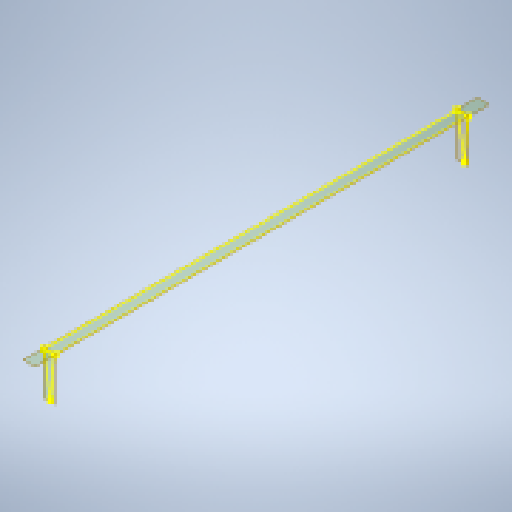
# Autodesk Inventor part: Aleiron
Saved by Autodesk Inventor 2026 (Build 300175050, 175E)
## iProperties
Created: 2025-07-28
Part Number: Aleiron
Material: Generic
Document SubType Name: Modeling
Designer: Cupri
Density: 1 g/cm^3
Appearance: Default
Author: Cupri
Autodesk Inventor part; units mm, degrees
ref_plane "YZ Plane" through (0, 0, 0) normal (1, 0, 0) x (0, 1, 0)
ref_plane "XZ Plane" through (0, 0, 0) normal (0, 1, 0) x (-1, 0, 0)
ref_plane "Work Plane1" through (0, 0, 0) normal (0, 0, 1) x (1, 0, 0)
sketch "Sketch1" plane through (0, 0, 0) normal (0, 0, 1) x (1, 0, 0)
  spline S0 degree 3 poles (-0.3432, 0) (-0.5476, 0.9305) (-1.8109, 6.8833) (-4.6379, 21.5083) (-5.8348, 28.0065) (-7.2785, 36.223) (-7.5554, 37.8163) (-8.144, 41.2441) (-8.4751, 43.1968) (-9.6001, 49.9214) (-10.403, 54.896) (-11.194, 60) knots -7.723672 -7.723672 -7.723672 -7.723672 -4.852573 -4.852573 -2.692004 -2.692004 -2.185384 -2.185384 -1.605169 -1.605169 -0.053083 -0.053083 -0.053083 -0.053083 projected
  spline S1 degree 3 poles (-0.3324, -0.0487) (-0.3358, -0.0335) (-0.3394, -0.0172) (-0.3432, 0) knots -0.056243 -0.056243 -0.056243 -0.056243 -0.050014 -0.050014 -0.050014 -0.050014 projected
  spline S2 degree 3 poles (0.4003, 0) (0.3914, -0.0334) (0.3779, -0.0655) (0.3429, -0.1252) (0.3214, -0.1525) (0.2602, -0.2119) (0.2174, -0.2397) (0.1233, -0.2774) (0.0729, -0.2868) (-0.0285, -0.2859) (-0.0786, -0.2756) (-0.1717, -0.2365) (-0.214, -0.2081) (-0.285, -0.1369) (-0.3131, -0.0949) (-0.3324, -0.0487) knots -0.096513 -0.096513 -0.096513 -0.096513 -0.086135 -0.086135 -0.075744 -0.075744 -0.060566 -0.060566 -0.045346 -0.045346 -0.030151 -0.030151 -0.015033 -0.015033 0 0 0 0 projected
  spline S3 degree 3 poles (4.5352, 60) (4.1492, 54.3024) (3.8851, 50.4553) (3.5768, 45.9572) (3.4952, 44.7719) (3.3704, 42.9615) (3.3433, 42.5677) (2.8933, 36.0424) (2.4653, 29.8794) (1.9678, 22.7306) (1.9176, 22.0094) (1.5419, 16.6071) (1.2042, 11.7834) (0.7423, 5.1029) (0.4375, 0.6896) (0.4003, 0) knots -1.505674 -1.505674 -1.505674 -1.505674 -1.330011 -1.330011 -1.237485 -1.237485 -1.213768 -1.213768 -0.810155 -0.810155 -0.745592 -0.745592 -0.207193 -0.207193 0 0 0 0 projected
  line L0 (-11.194, 60) -> (4.5352, 60) projected
  point P0 (0, 0)
ref_plane "Work Plane2" through (-0.5511, 59.985, 603.2266) normal (-0.0007, 0, -1) x (-1, 0.0063, 0.0007)
sketch "Sketch2" plane through (-0.5511, 59.985, 603.2266) normal (-0.0007, 0, -1) x (-1, 0.0063, 0.0007)
  spline S0 degree 3 poles (10.5494, 0) (10.2293, -2.2481) (9.8995, -4.4964) (9.1887, -9.2246) (8.8031, -11.7217) (7.617, -19.2349) (6.7636, -24.413) (5.6798, -30.7739) (5.4357, -32.1924) (4.488, -37.646) (3.7345, -41.8662) (1.487, -53.9406) (0.6091, -57.9871) (0.1466, -60) knots -1.758139 -1.758139 -1.758139 -1.758139 -1.591949 -1.591949 -1.406575 -1.406575 -1.02993 -1.02993 -0.92277 -0.92277 -0.615604 -0.615604 -0.003901 -0.003901 -0.003901 -0.003901 projected
  line L0 (-4.5586, 0) -> (10.5494, 0) projected
  spline S1 degree 3 poles (-0.4384, -60) (-0.5115, -58.4166) (-0.6219, -56.3988) (-0.8889, -51.9428) (-1.0365, -49.6525) (-1.4591, -43.3117) (-1.7767, -38.8185) (-2.2573, -32.1106) (-2.4709, -29.16) (-2.7817, -24.8733) (-2.8913, -23.3626) (-3.3521, -17.0005) (-3.6389, -13.0261) (-3.987, -8.1315) (-4.0258, -7.5846) (-4.2301, -4.7006) (-4.3955, -2.346) (-4.5586, 0) knots -6.638256 -6.638256 -6.638256 -6.638256 -5.879486 -5.879486 -5.125599 -5.125599 -3.729436 -3.729436 -2.742881 -2.742881 -2.242014 -2.242014 -0.922307 -0.922307 -0.757416 -0.757416 -0.052368 -0.052368 -0.052368 -0.052368 projected
  spline S2 degree 3 poles (0.1378, -60.0383) (0.1276, -60.0613) (0.1145, -60.083) (0.0834, -60.1227) (0.0654, -60.1405) (0.0137, -60.1806) (-0.0226, -60.1987) (-0.1, -60.22) (-0.1405, -60.223) (-0.2203, -60.2134) (-0.2588, -60.2008) (-0.3286, -60.1618) (-0.3593, -60.1358) (-0.4088, -60.0736) (-0.4273, -60.0381) (-0.4384, -60) knots -0.075123 -0.075123 -0.075123 -0.075123 -0.067561 -0.067561 -0.059991 -0.059991 -0.047948 -0.047948 -0.035886 -0.035886 -0.023859 -0.023859 -0.011899 -0.011899 0 0 0 0 projected
  spline S3 degree 3 poles (0.1466, -60) (0.1437, -60.0128) (0.1407, -60.0255) (0.1378, -60.0383) knots -0.00392 -0.00392 -0.00392 -0.00392 0 0 0 0 projected
  point P0 (-1.322, -59.9791)
ref_plane "Work Plane3" through (0, 60, 0) normal (0, -1, 0) x (-1, 0, 0)
sketch "Sketch3" plane through (0, 60, 0) normal (0, -1, 0) x (-1, 0, 0)
  line L0 (-4.5585, -602.272) -> (10.5506, -602.272) projected
  spline S0 degree 3 poles (11.194, 0) (11.0061, -196.1225) (10.7842, -410.86) (10.5506, -602.272) knots -57.533814 -57.533814 -57.533814 -57.533814 -0.145819 -0.145819 -0.145819 -0.145819 projected
  line L1 (11.194, 0) -> (-4.5352, 0) projected
  spline S1 degree 3 poles (-4.5585, -602.272) (-4.5373, -395.7385) (-4.5305, -201.8279) (-4.5352, 0) knots -60.602558 -60.602558 -60.602558 -60.602558 -0.050245 -0.050245 -0.050245 -0.050245 projected
  point P0 (0, 0)
ref_plane "Work Plane4" through (0, 0, 0) normal (0, 0, 1) x (1, 0, 0)
sketch "Sketch4" plane through (0, 0, 0) normal (0, 0, 1) x (1, 0, 0)
  spline S0 degree 3 poles (-0.3432, 0) (-0.5476, 0.9305) (-1.8109, 6.8833) (-4.6379, 21.5083) (-5.8348, 28.0065) (-7.2785, 36.223) (-7.5554, 37.8163) (-8.144, 41.2441) (-8.4751, 43.1968) (-9.6001, 49.9214) (-10.403, 54.896) (-11.194, 60) knots -7.723672 -7.723672 -7.723672 -7.723672 -4.852573 -4.852573 -2.692004 -2.692004 -2.185384 -2.185384 -1.605169 -1.605169 -0.053083 -0.053083 -0.053083 -0.053083 projected
  spline S1 degree 3 poles (-0.3324, -0.0487) (-0.3358, -0.0335) (-0.3394, -0.0172) (-0.3432, 0) knots -0.056243 -0.056243 -0.056243 -0.056243 -0.050014 -0.050014 -0.050014 -0.050014 projected
  spline S2 degree 3 poles (0.4003, 0) (0.3914, -0.0334) (0.3779, -0.0655) (0.3429, -0.1252) (0.3214, -0.1525) (0.2602, -0.2119) (0.2174, -0.2397) (0.1233, -0.2774) (0.0729, -0.2868) (-0.0285, -0.2859) (-0.0786, -0.2756) (-0.1717, -0.2365) (-0.214, -0.2081) (-0.285, -0.1369) (-0.3131, -0.0949) (-0.3324, -0.0487) knots -0.096513 -0.096513 -0.096513 -0.096513 -0.086135 -0.086135 -0.075744 -0.075744 -0.060566 -0.060566 -0.045346 -0.045346 -0.030151 -0.030151 -0.015033 -0.015033 0 0 0 0 projected
  spline S3 degree 3 poles (4.5352, 60) (4.1492, 54.3024) (3.8851, 50.4553) (3.5768, 45.9572) (3.4952, 44.7719) (3.3704, 42.9615) (3.3433, 42.5677) (2.8933, 36.0424) (2.4653, 29.8794) (1.9678, 22.7306) (1.9176, 22.0094) (1.5419, 16.6071) (1.2042, 11.7834) (0.7423, 5.1029) (0.4375, 0.6896) (0.4003, 0) knots -1.505674 -1.505674 -1.505674 -1.505674 -1.330011 -1.330011 -1.237485 -1.237485 -1.213768 -1.213768 -0.810155 -0.810155 -0.745592 -0.745592 -0.207193 -0.207193 0 0 0 0 projected
  line L0 (-11.194, 60) -> (4.5352, 60) projected
  point P0 (0, 0)
ref_plane "Work Plane5" through (-11.4796, -0.2671, 603.2336) normal (-0.0007, 0, -1) x (0.0063, 1, 0)
extrude "Extrusion1" add sketch "Sketch4" along normal up to surface (603.2261 mm away)
fillet "Fillet1" radius 6.35 2 edges at (-11.194, 60, 301.6131) (4.5352, 60, 301.6131)
body "Solid1"
